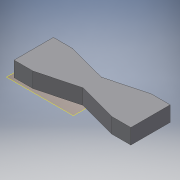
# Autodesk Inventor part: Bow Tie Key
Saved by Autodesk Inventor 2017 (Build 210142000, 142)
## iProperties
Created: 2017-03-25
Part Number: Bow Tie Key
Material: Generic
Document SubType Name: Modeling
Designer: Diego
Density: 1 g/cm^3
Appearance: Default
Author: Diego
Autodesk Inventor part; units mm, degrees
ref_plane "YZ Plane" through (0, 0, 0) normal (1, 0, 0) x (0, 1, 0)
ref_plane "XZ Plane" through (0, 0, 0) normal (0, 1, 0) x (-1, 0, 0)
ref_plane "XY Plane" through (0, 0, 0) normal (0, 0, 1) x (1, 0, 0)
ref_plane "Work Plane1" through (0, 0, 0) normal (0, 0, 1) x (1, 0, 0)
sketch "Sketch1" plane through (0, 0, 0) normal (0, 0, 1) x (1, 0, 0)
  line L0 (-1.6732, -5.15) -> (-6.6732, -5.15) projected
  line L1 (8.3268, -2.5) -> (-1.6732, -5.15) projected
  line L2 (8.3268, 2.5) -> (8.3268, -2.5) projected
  line L3 (-1.6732, 5.15) -> (8.3268, 2.5) projected
  line L4 (-6.6732, 5.15) -> (-1.6732, 5.15) projected
  line L5 (-6.6732, -5.15) -> (-6.6732, 5.15) projected
  line L6 (-1.7123, -4.85) -> (-6.3732, -4.85)
  line L7 (-6.3732, -4.85) -> (-6.3732, 4.85)
  line L8 (-6.3732, 4.85) -> (-1.7123, 4.85)
  line L9 (-1.7123, 4.85) -> (8.0268, 2.2691)
  line L10 (8.0268, 2.2691) -> (8.0268, -2.2691)
  line L11 (8.0268, -2.2691) -> (-1.7123, -4.85)
  point P0 (0, 0)
  dimension "d0" = 0.3
  constraints: 12 end point, 5 other
  measures "d0" distance between parallel lines of L1 L11
ref_plane "Work Plane2" through (-1.6732, 2.5, 3.75) normal (0, 0, 1) x (1, 0, 0)
extrude "Extrusion1" add sketch "Sketch1" along normal up to surface (3.75 mm away) contours L6 L7 L8 L9 L10 L11
mirror "Mirror1" about plane through (8.0268, -2.2691, 0) normal (1, 0, 0) of "Extrusion1"
body "Solid1"
